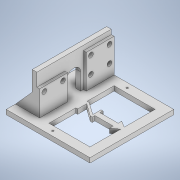
# Autodesk Inventor part: HallSensor_Halterung
Saved by Autodesk Inventor 2022.2 (Build 262287010, 287A)
## iProperties
Created: 2024-01-10
Part Number: HallSensor_Halterung
Material: Generisch
Document SubType Name: Modeling
Designer: ppovolni
Density: 1 g/cm^3
Appearance: Vorgabe
Author: ppovolni
Autodesk Inventor part; units mm, degrees
ref_plane "Arbeitsebene2" through (-75, 27.1, 0) normal (0, 0, 1) x (0, 1, 0)
sketch "center1" plane through (-75, 27.1, 0) normal (0, 0, 1) x (0, 1, 0)
  line L0 (-173.891, -75) -> (168.1592, -75)
  line L1 (0, 344.1359) -> (0, -385.7952)
  point P0 (-27.1, -75)
  constraints: 4 end point, 1 horizontal, 1 vertical, 4 other
ref_plane "Arbeitsebene3" through (0, 99.4, -2.4) normal (-1, 0, 0) x (0, 0, 1)
sketch "center2" plane through (0, 99.4, -2.4) normal (-1, 0, 0) x (0, 0, 1)
  line L0 (184.8129, -72.3) -> (-258.9785, -72.3)
  point P0 (2.4, -99.4)
  constraints: 2 end point, 1 horizontal, 2 other
sketch "Groundplane" plane through (0, 0, 0) normal (0, 1, 0) x (-1, 0, 0)
  line L0 (45, 45) -> (-45, 45) construction
  line L1 (-45, 45) -> (-45, -45) construction
  line L2 (-45, -45) -> (45, -45) construction
  line L3 (45, -45) -> (45, 45) construction
  line L4 (1, 45) -> (-1, 45) construction
  line L5 (-1, 45) -> (-1, 40) construction
  line L6 (-1, 40) -> (1, 40) construction
  line L7 (1, 40) -> (1, 45) construction
  arc A0 (-1, 40) -> (1, 40) centre (0, 40) ccw construction
  line L8 (1, -45) -> (-1, -45) construction
  line L9 (-1, -45) -> (-1, -40) construction
  line L10 (-1, -40) -> (1, -40) construction
  line L11 (1, -40) -> (1, -45) construction
  arc A1 (1, -40) -> (-1, -40) centre (0, -40) ccw construction
  line L12 (0, -350.1368) -> (0, 271.1712) projected
  point P0 (0, 0)
  point P1 (0, -45)
  dimension "d5" = 2
  dimension "d6" = 5
  dimension "d7" = 2
  dimension "d8" = 5
  dimension "d9" = 90
  dimension "d63" = 90
  dimension "d76" = 45
  constraints: 24 end point, 6 parallel, 4 point on circle, 4 point on line, 3 horizontal, 3 perpendicular, 2 centre point, 2 midpoint, 2 tangent, 1 vertical alignment
  measures "d5" distance between parallel lines of L5 L7
  measures "d6" distance of L4.end L5.end
  measures "d7" distance between parallel lines of L9 L11
  measures "d8" distance of L8.end L9.end
  measures "d9" distance of L2.end L0.start
  measures "d63" distance of L1.end L2.end
  measures "d76" distance from line of L0 point (0, 0)
sketch "Hallsensor" plane through (0, 0, 0) normal (1, 0, 0) x (0, 1, 0)
  line L0 (22.1, 0) -> (32.1, 0) construction
  line L1 (32.1, 0) -> (32.1, 20) construction
  line L2 (32.1, 20) -> (22.1, 20) construction
  line L3 (22.1, 20) -> (22.1, 0) construction
  line L4 (27.1, 182.4129) -> (27.1, -261.3785) construction
  line L5 (-146.791, 0) -> (195.2592, 0) construction
  line L6 (31.1, 1) -> (33.1, 1)
  line L7 (33.1, 1) -> (33.1, -1)
  line L8 (33.1, -1) -> (31.1, -1)
  line L9 (31.1, -1) -> (31.1, 1)
  line L10 (31.1, 1) -> (33.1, -1) construction
  line L11 (33.1, 1) -> (31.1, -1) construction
  line L12 (21.1, 1) -> (23.1, 1)
  line L13 (23.1, 1) -> (23.1, -1)
  line L14 (23.1, -1) -> (21.1, -1)
  line L15 (21.1, -1) -> (21.1, 1)
  line L16 (21.1, 1) -> (23.1, -1) construction
  line L17 (23.1, 1) -> (21.1, -1) construction
  line L18 (31.1, 21) -> (33.1, 21)
  line L19 (33.1, 21) -> (33.1, 19)
  line L20 (33.1, 19) -> (31.1, 19)
  line L21 (31.1, 19) -> (31.1, 21)
  line L22 (31.1, 21) -> (33.1, 19) construction
  line L23 (33.1, 21) -> (31.1, 19) construction
  line L24 (21.1, 21) -> (23.1, 21)
  line L25 (23.1, 21) -> (23.1, 19)
  line L26 (23.1, 19) -> (21.1, 19)
  line L27 (21.1, 19) -> (21.1, 21)
  line L28 (21.1, 21) -> (23.1, 19) construction
  line L29 (23.1, 21) -> (21.1, 19) construction
  line L30 (36.1, 30) -> (18.1, 30) construction
  line L31 (18.1, 30) -> (18.1, -20) construction
  line L32 (18.1, -20) -> (36.1, -20) construction
  line L33 (36.1, -20) -> (36.1, 30) construction
  circle A0 centre (27.1, 30) radius 1.6
  circle A1 centre (36.1, -20) radius 1.6
  circle A2 centre (18.1, -20) radius 1.6
  point P0 (0, 0)
  dimension "d127" = 20
  dimension "d128" = 5
  dimension "d129" = 5
  dimension "d130" = 2
  dimension "d131" = 20
  dimension "d132" = 4
  dimension "d133" = 4
  dimension "d134" = 10
  dimension "d135" = 3.2
  constraints: 64 end point, 12 parallel, 9 midpoint, 6 horizontal, 6 perpendicular, 5 equal length, 3 centre point, 2 coincident, 2 equal radius, 2 point on line, 1 collinear
  measures "d127" distance of L0.end L1.end
  measures "d128" distance between parallel lines of L4 L1
  measures "d129" distance between parallel lines of L3 L4
  measures "d130" distance of L18.end L19.end
  measures "d131" distance between parallel lines of L0 L32
  measures "d132" distance between parallel lines of L1 L33
  measures "d133" distance between parallel lines of L31 L3
  measures "d134" distance between parallel lines of L30 L2
  measures "d135" diameter of A0
ref_plane "Arbeitsebene1" through (-27.1, 0, 0) normal (1, 0, 0) x (0, 1, 0)
sketch "Montagepunkte" plane through (-27.1, 0, 0) normal (1, 0, 0) x (0, 1, 0)
  line L0 (27.1, 10) -> (27.1, -45.0561) construction
  line L1 (46.1, -45) -> (0, -45)
  line L2 (0, -45) -> (0, 35)
  line L3 (0, 35) -> (46.1, 35)
  line L4 (46.1, 35) -> (46.1, -45)
  circle A0 centre (36.1, -20) radius 1.6 projected
  circle A1 centre (18.1, -20) radius 1.6 projected
  circle A2 centre (27.1, 30) radius 1.6 projected
  line L5 (36.1, -20) -> (18.1, -20) construction
  line L6 (18.1, -20) -> (18.1, -40) construction
  line L7 (18.1, -40) -> (36.1, -40) construction
  line L8 (36.1, -40) -> (36.1, -20) construction
  line L9 (27.1, 30) -> (27.1, 10) construction
  circle A3 centre (27.1, 10) radius 1.6
  circle A4 centre (36.1, -40) radius 1.6
  circle A5 centre (18.1, -40) radius 1.6
  point P0 (0, 0)
  point P1 (0, 0)
  point P2 (1.45, 0)
  dimension "d136" = 20
  dimension "d137" = 20
  dimension "d138" = 3.2
  dimension "d139" = 5
  dimension "d140" = 5
  dimension "d141" = 10
  constraints: 20 end point, 4 parallel, 3 centre point, 3 coincident, 2 equal radius, 2 horizontal, 2 perpendicular, 2 point on line, 2 vertical
  measures "d136" distance between parallel lines of L7 L5
  measures "d137" distance of L9.start L9.end
  measures "d138" diameter of A4
  measures "d139" distance from line of L3 L9.start
  measures "d140" distance from line of L1 L7.end
  measures "d141" distance from line of L4 L7.end
sketch "Skizze10" plane through (-27.1, 0, 0) normal (1, 0, 0) x (0, 1, 0)
  line L0 (46.1, -45) -> (0, -45) projected
  line L1 (0, -45) -> (0, 35) projected
  line L2 (0, 35) -> (46.1, 35) projected
  line L3 (46.1, 35) -> (46.1, -45) projected
  point P0 (0, 0)
extrude "Extrusion5" add sketch "Skizze10" along normal blind 5
sketch "Skizze11" plane through (-22.1, 0, 0) normal (1, 0, 0) x (0, 0, -1)
  line L0 (-35, 0) -> (45, 0) projected
  circle A0 centre (40, 36.1) radius 1.6 projected
  circle A1 centre (20, 36.1) radius 1.6 projected
  circle A2 centre (20, 18.1) radius 1.6 projected
  circle A3 centre (40, 18.1) radius 1.6 projected
  circle A4 centre (-10, 27.1) radius 1.6 projected
  circle A5 centre (-30, 27.1) radius 1.6 projected
  line L1 (-35, 32.1) -> (-5, 32.1)
  line L2 (-5, 32.1) -> (-5, 0)
  line L3 (-5, 0) -> (-35, 0)
  line L4 (-35, 0) -> (-35, 32.1)
  line L5 (15, 41.1) -> (45, 41.1)
  line L6 (45, 41.1) -> (45, 0)
  line L7 (45, 0) -> (15, 0)
  line L8 (15, 0) -> (15, 41.1)
  point P0 (0, 0)
  dimension "d142" = 5
  dimension "d143" = 5
  dimension "d144" = 5
  dimension "d145" = 5
  dimension "d146" = 5
  dimension "d147" = 5
  constraints: 16 end point, 4 parallel, 2 horizontal, 2 perpendicular, 2 point on line
  measures "d142" distance from line of L1 A4.centre
  measures "d143" distance from line of L2 A4.centre
  measures "d144" distance from line of L4 A5.centre
  measures "d145" distance from line of A0.centre L6
  measures "d146" distance from line of A1.centre L5
  measures "d147" distance from line of L8 A1.centre
extrude "Extrusion6" add sketch "Skizze11" along normal blind 3
chamfer "Fase3" distance 1 distance2 3 4 edges at (-19.1, 36.1, -18.4) (-19.1, 36.1, -38.4) (-19.1, 18.1, -38.4) (-19.1, 18.1, -18.4) measured on face at (-19.1, 5.5944, -26.9696)
chamfer "Fase4" distance 1 distance2 3 2 edges at (-19.1, 27.1, 31.6) (-19.1, 27.1, 11.6) measured on face at (-19.1, 8.5944, 16.9696)
sketch "Skizze12" plane through (0, 0, 0) normal (0, 1, 0) x (-1, 0, 0)
  line L0 (-45, 45) -> (-45, -45) construction
  line L1 (-45, -45) -> (45, -45) construction
  line L2 (45, -45) -> (45, 45) construction
  line L3 (45, 45) -> (-45, 45) construction
  arc A0 (1, -40) -> (-1, -40) centre (0, -40) ccw construction
  arc A1 (-1, 40) -> (1, 40) centre (0, 40) ccw construction
  circle A2 centre (0, 40) radius 1
  circle A3 centre (0, -40) radius 1
  line L4 (45, -45) -> (-45, -45)
  line L5 (-45, -45) -> (-45, 45)
  line L6 (-45, 45) -> (45, 45)
  line L7 (45, 45) -> (45, -45)
  point P0 (0, 0)
  constraints: 8 end point, 2 coincident, 2 horizontal alignment, 2 parallel, 1 horizontal, 1 perpendicular, 5 other
extrude "Extrusion7" add sketch "Skizze12" along normal blind 5
sketch "Skizze13" plane through (-27.1, 46.1, 35) normal (0, 0, 1) x (1, 0, 0)
  line L0 (0, -21.1) -> (-17.9, -41.1)
  line L1 (-17.9, -41.1) -> (0, -41.1)
  line L2 (0, -41.1) -> (0, -21.1)
  point P0 (27.1, -46.1)
  dimension "d108" = 20
  constraints: 6 end point, 1 coincident, 1 horizontal, 1 perpendicular
  measures "d108" distance of L1.end L0.start
extrude "Extrusion8" add sketch "Skizze13" against normal blind 5
sketch "Skizze14" plane through (-19.1, 46.1, -45) normal (0, 0, -1) x (-1, 0, 0)
  line L0 (25.9, -41.1) -> (8, -41.1) projected
  line L1 (25.9, -41.1) -> (8, -21.1) projected
  line L2 (8, -41.1) -> (8, -21.1) projected
  point P0 (-19.1, -46.1)
extrude "Extrusion9" add sketch "Skizze14" against normal blind 5
sketch "Skizze15" plane through (-27.1, 0, 0) normal (-1, 0, 0) x (0, 0, 1)
  line L0 (-12, 5) -> (3, 5)
  line L1 (3, 5) -> (3, 23)
  line L2 (-4, 30) -> (-5, 30)
  line L3 (-12, 23) -> (-12, 5)
  line L4 (-45, 5) -> (35, 5) projected
  arc A0 (-5, 30) -> (-12, 23) centre (-5, 23) ccw
  arc A1 (3, 23) -> (-4, 30) centre (-4, 23) ccw
  point P0 (0, 0)
  point P1 (3, 30)
  point P2 (-12, 30)
  point P3 (-40, 5)
  point P4 (30, 5)
  dimension "d114" = 15
  dimension "d115" = 25
  dimension "d116" = 7
  constraints: 8 end point, 4 point on circle, 4 point on line, 4 tangent, 2 centre point, 2 parallel, 1 collinear, 1 equal radius, 1 horizontal, 1 perpendicular
  measures "d114" distance of point (3, 30) point (-12, 30)
  measures "d115" distance of point (-12, 30) L0.start
  measures "d116" radius of A0
extrude "Extrusion10" cut sketch "Skizze15" against normal through all
sketch "Skizze16" plane through (0, 5, 0) normal (0, 1, 0) x (1, 0, 0)
  line L0 (-9.1, 35) -> (35, 35)
  line L1 (35, 35) -> (35, -35)
  line L2 (35, -35) -> (-9.1, -35)
  line L3 (-9.1, -35) -> (-9.1, 35)
  line L4 (45, 45) -> (-19.1, 45) projected
  line L5 (45, -45) -> (45, 45) projected
  line L6 (-45, -45) -> (45, -45) projected
  line L7 (-19.1, -35) -> (-19.1, -5) construction
  point P0 (0, 0)
  dimension "d119" = 10
  dimension "d120" = 10
  dimension "d121" = 10
  dimension "d148" = 10
  constraints: 8 end point, 2 parallel, 1 horizontal, 1 perpendicular
  measures "d119" distance between parallel lines of L0 L4
  measures "d120" distance between parallel lines of L5 L1
  measures "d121" distance between parallel lines of L6 L2
  measures "d148" distance between parallel lines of L3 L7
extrude "Extrusion11" cut sketch "Skizze16" against normal through all
sketch "Skizze17" plane through (-45, 0, 45) normal (0, -1, 0) x (1, 0, 0)
  line L0 (35.9, -80) -> (35.9, -10) construction
  line L1 (83, -45) -> (73, -51.0852)
  line L2 (73, -51.0852) -> (73, -47.2557)
  line L3 (73, -47.2557) -> (53, -47.2557)
  line L4 (53, -47.2557) -> (53, -41.9148)
  line L5 (53, -41.9148) -> (73, -41.9148)
  line L6 (73, -41.9148) -> (73, -38.0852)
  line L7 (73, -38.0852) -> (83, -45)
  line L8 (-520.1221, -45) -> (501.7814, -45) projected
  line L9 (35.9, -38.7956) -> (35.9, -51.0201)
  line L10 (35.9, -51.0201) -> (38.0698, -51.0201)
  line L11 (38.0698, -51.0201) -> (51.3295, -41.6603)
  line L12 (51.3295, -41.6603) -> (51.3295, -50.5946)
  line L13 (51.3295, -50.5946) -> (53.4, -50.5946)
  line L14 (53.4, -50.5946) -> (53.4, -39.0367)
  line L15 (53.4, -39.0367) -> (51.3011, -39.0367)
  line L16 (51.3011, -39.0367) -> (37.9705, -48.4957)
  line L17 (37.9705, -48.4957) -> (37.9705, -38.7956)
  line L18 (37.9705, -38.7956) -> (35.9, -38.7956)
  point P0 (45, -45)
  constraints: 15 end point, 3 perpendicular, 3 point on line, 2 vertical, 1 collinear
extrude "Extrusion12" add sketch "Skizze17" against normal up to surface (5 mm away) contours L8 L14 L5 L6 L7 | L1 L2 L3 L14 L8 | L14 L3 L4 L8 | L8 L4 L5 L14 | L8 L12 L11 L16 L15 L14 L5 L4 | L4 L3 L14 L13 L12 L8 | L11 L10 L9 L8 L17 L16 | L8 L9 L18 L17
